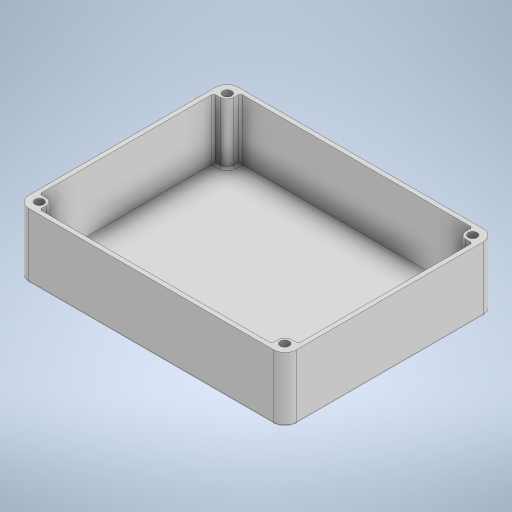
# Autodesk Inventor part: Boitier_aluminium
Saved by Autodesk Inventor 2024 (Build 280153000, 153)
## iProperties
Created: 2024-08-29
Part Number: Boitier_aluminium
Material: Générique
Document SubType Name: Modeling
Designer: malam
Density: 1 g/cm^3
Appearance: Par défaut
Author: malam
Autodesk Inventor part; units mm, degrees
ref_plane "YZ Plane" through (0, 0, 0) normal (1, 0, 0) x (0, 1, 0)
ref_plane "XZ Plane" through (0, 0, 0) normal (0, 1, 0) x (-1, 0, 0)
ref_plane "XY Plane" through (0, 0, 0) normal (0, 0, 1) x (1, 0, 0)
sketch "Esquisse1" plane through (0, 0, 0) normal (0, 1, 0) x (-1, 0, 0)
  line L0 (60, 47) -> (-60, 47)
  line L1 (-60, 47) -> (-60, -47)
  line L2 (-60, -47) -> (60, -47)
  line L3 (60, -47) -> (60, 47)
  line L4 (60, 47) -> (-60, -47) construction
  line L5 (-60, 47) -> (60, -47) construction
  line L6 (60, -47) -> (52, -47)
  line L7 (52, -47) -> (52, -39)
  line L8 (52, -39) -> (60, -39)
  line L9 (60, -39) -> (60, -47)
  line L10 (-60, -47) -> (-52, -47)
  line L11 (-52, -47) -> (-52, -39)
  line L12 (-52, -39) -> (-60, -39)
  line L13 (-60, -39) -> (-60, -47)
  line L14 (60, 47) -> (52, 47)
  line L15 (52, 47) -> (52, 39)
  line L16 (52, 39) -> (60, 39)
  line L17 (60, 39) -> (60, 47)
  line L18 (-60, 47) -> (-52, 47)
  line L19 (-52, 47) -> (-52, 39)
  line L20 (-52, 39) -> (-60, 39)
  line L21 (-60, 39) -> (-60, 47)
  circle A0 centre (-55, -42.115) radius 2
  line L22 (0, -47.6968) -> (0, 50.167) construction
  line L23 (81.8074, 0) -> (-86.221, 0) construction
  circle A1 centre (55, -42.115) radius 2
  circle A2 centre (-55, 42.115) radius 2
  circle A3 centre (55, 42.115) radius 2
  line L24 (58, -47) -> (58, 47)
  line L25 (60, 45) -> (-60, 45)
  line L26 (-60, -45) -> (60, -45)
  line L27 (-58, -47) -> (-58, 47)
  point P0 (0, 0)
  point P1 (-58, 39)
  point P2 (-58, -39)
  point P3 (-52, -45)
  point P4 (52, -45)
  point P5 (58, -39)
  point P6 (58, 39)
  point P7 (52, 45)
  point P8 (-52, 45)
  dimension "d0" = 120
  dimension "d1" = 94
  dimension "d2" = 8
  dimension "d3" = 8
  dimension "d4" = 8
  dimension "d5" = 8
  dimension "d6" = 8
  dimension "d8" = 4
  dimension "d9" = 55
  dimension "d10" = 42.115
  dimension "d11" = 8
  dimension "d12" = 2
  dimension "d13" = 2
  dimension "d14" = 2
  dimension "d15" = 2
  constraints: 56 end point, 10 parallel, 10 point on line, 9 perpendicular, 6 horizontal, 4 centre point, 3 symmetric about line, 2 midpoint, 1 vertical, 3 other
  measures "d0" distance of L2.end L1.end
  measures "d1" distance of L1.end L0.end
  measures "d2" distance of L7.end L8.end
  measures "d3" distance of L6.end L7.end
  measures "d4" distance of L12.end L11.end
  measures "d5" distance of L15.end L14.end
  measures "d6" distance of L18.end L19.end
  measures "d8" diameter of A0
  measures "d9" distance from line of A0.centre L22
  measures "d10" distance from line of L23 A0.centre
  measures "d11" distance of L19.end L20.end
  measures "d12" distance between parallel lines of L3 L24
  measures "d13" distance between parallel lines of L2 L26
  measures "d14" distance between parallel lines of L1 L27
  measures "d15" distance between parallel lines of L0 L25
extrude "Extrusion1" add sketch "Esquisse1" along normal blind 2 contours L15 L16 L24 L8 L7 L26 L11 L12 L27 L20 L19 L25
extrude "Extrusion2" add sketch "Esquisse1" along normal blind 29.1 contours L3 L25 L24 L0 | L24 L25 L15 L0 | L3 L16 L24 L25 | L15 L25 L19 L0 | L24 L16 L15 L25 | L3 L8 L24 L16 | L19 L25 L27 L0 | L3 L26 L24 L8 | L27 L25 L1 L0 | L19 L20 L27 L25 | L24 L26 L7 L8 | L3 L2 L24 L26 | L27 L20 L1 L25 | L24 L2 L7 L26 | L27 L12 L1 L20 | L7 L2 L11 L26 | L27 L26 L1 L12 | L12 L11 L26 L27 | L11 L2 L27 L26 | L27 L2 L1 L26
fillet "Congé1" radius 5 4 edges at (-60, 14.55, 47) (-60, 14.55, -47) (60, 14.55, -47) (60, 14.55, 47)
fillet "Congé2" radius 3 4 edges at (-52, 15.55, -39) (-52, 15.55, 39) (52, 15.55, -39) (52, 15.55, 39)
fillet "Congé3" radius 1 16 edges at (-58, 15.55, -39) (-52, 15.55, -45) (-52, 2, -43.5) (-56.5, 2, -39) (56.5, 2, -39) (52, 2, -43.5) (52, 15.55, -45) (58, 15.55, -39) (58, 15.55, 39) (52, 15.55, 45) (52, 2, 43.5) (56.5, 2, 39) (-56.5, 2, 39) (-52, 2, 43.5) (-58, 15.55, 39) (-52, 15.55, 45)
extrude "Extrusion3" add sketch "Esquisse1" along normal blind 19.1 contours A0 | A1 | A2 | A3
thread "Filetage1" size "M4x0.7" class "6H" standard "ANSI Metric M Profile" length 40
thread "Filetage2" size "M4x0.7" class "6H" standard "ANSI Metric M Profile" length 40
thread "Filetage3" size "M4x0.7" class "6H" standard "ANSI Metric M Profile" length 40
thread "Filetage4" size "M4x0.7" class "6H" standard "ANSI Metric M Profile" length 40
fillet "Congé4" radius 1 4 edges at (0, 0, 47) (60, 0, 0) (0, 0, -47) (-60, 0, 0)
sketch "Esquisse2" plane through (0, 29.1, 0) normal (0, 1, 0) x (1, 0, 0)
  arc A0 (55, -47) -> (60, -42) centre (55, -42) ccw projected
  line L0 (60, -42) -> (60, 42) projected
  arc A1 (60, 42) -> (55, 47) centre (55, 42) ccw projected
  line L1 (55, 47) -> (-55, 47) projected
  arc A2 (-55, 47) -> (-60, 42) centre (-55, 42) ccw projected
  line L2 (-60, 42) -> (-60, -42) projected
  arc A3 (-60, -42) -> (-55, -47) centre (-55, -42) ccw projected
  line L3 (-55, -47) -> (55, -47) projected
  circle A4 centre (55, 42.115) radius 2 projected
  circle A5 centre (55, -42.115) radius 2 projected
  circle A6 centre (-55, 42.115) radius 2 projected
  circle A7 centre (-55, -42.115) radius 2 projected
  arc A8 (55, -39) -> (52, -42) centre (55, -42) ccw projected
  line L4 (52, -42) -> (52, -44) projected
  arc A9 (51, -45) -> (52, -44) centre (51, -44) ccw projected
  line L5 (51, -45) -> (-51, -45) projected
  arc A10 (-52, -44) -> (-51, -45) centre (-51, -44) ccw projected
  line L6 (-52, -44) -> (-52, -42) projected
  arc A11 (-52, -42) -> (-55, -39) centre (-55, -42) ccw projected
  line L7 (-55, -39) -> (-57, -39) projected
  arc A12 (-58, -38) -> (-57, -39) centre (-57, -38) ccw projected
  line L8 (-58, -38) -> (-58, 38) projected
  arc A13 (-57, 39) -> (-58, 38) centre (-57, 38) ccw projected
  line L9 (-57, 39) -> (-55, 39) projected
  arc A14 (-55, 39) -> (-52, 42) centre (-55, 42) ccw projected
  line L10 (-52, 42) -> (-52, 44) projected
  arc A15 (-51, 45) -> (-52, 44) centre (-51, 44) ccw projected
  line L11 (-51, 45) -> (51, 45) projected
  arc A16 (52, 44) -> (51, 45) centre (51, 44) ccw projected
  line L12 (52, 44) -> (52, 42) projected
  arc A17 (52, 42) -> (55, 39) centre (55, 42) ccw projected
  line L13 (55, 39) -> (57, 39) projected
  arc A18 (58, 38) -> (57, 39) centre (57, 38) ccw projected
  line L14 (58, 38) -> (58, -38) projected
  arc A19 (57, -39) -> (58, -38) centre (57, -38) ccw projected
  line L15 (57, -39) -> (55, -39) projected
  point P0 (0, 0)
